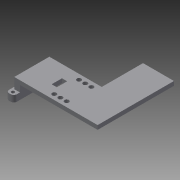
# Autodesk Inventor part: CartServoMountV2
Saved by Autodesk Inventor 2015 (Build 190159000, 159)
## iProperties
Created: 2016-03-28
Part Number: CartServoMountV2
Material: Generic
Document SubType Name: Modeling
Designer: Hatch
Density: 1 g/cm^3
Appearance: Default
Author: Hatch
Autodesk Inventor part; units mm, degrees
ref_plane "YZ Plane" through (0, 0, 0) normal (1, 0, 0) x (0, 1, 0)
ref_plane "XZ Plane" through (0, 0, 0) normal (0, 1, 0) x (-1, 0, 0)
ref_plane "XY Plane" through (0, 0, 0) normal (0, 0, 1) x (1, 0, 0)
sketch "Sketch1" plane through (0, 0, 0) normal (0, 1, 0) x (-1, 0, 0)
  line L0 (0, 0) -> (22, 0)
  line L1 (22, 0) -> (22, -34)
  line L2 (22, -34) -> (0, -34)
  line L3 (0, -34) -> (0, 0)
  dimension "d0" = 22
  dimension "d1" = 34
  constraints: 8 end point, 2 parallel, 1 horizontal, 1 perpendicular
  measures "d0" distance of L1.end L2.end
  measures "d1" distance of L0.end L1.end
extrude "Extrusion1" add sketch "Sketch1" along normal blind 4
sketch "Sketch2" plane through (0, 4, 0) normal (0, 1, 0) x (1, 0, 0)
  line L0 (-22, 0) -> (0, 0) projected
  circle A0 centre (-5, 5) radius 2.125
  dimension "d7" = 4.25
  constraints: 1 centre point
  measures "d7" diameter of A0
extrude "Extrusion2" cut sketch "Sketch2" against normal through all
pattern_linear "Rectangular Pattern1" count 3 spacing 6 along (-1, 0, 0) count 2 spacing 24 along (0, 0, -1) of "Extrusion2"
sketch "Sketch3" plane through (-22, 0, -34) normal (-1, 0, 0) x (0, 0, 1)
  line L0 (34, 0) -> (0, 0)
  line L1 (0, 0) -> (0, 4)
  line L2 (0, 4) -> (34, 4)
  line L3 (34, 4) -> (34, 0)
  constraints: 8 end point, 2 parallel, 1 horizontal, 1 perpendicular
extrude "Extrusion3" add sketch "Sketch3" along normal blind 23.25
sketch "Sketch4" plane through (0, 4, 0) normal (0, 1, 0) x (1, 0, 0)
  line L0 (-45.25, 0) -> (-50.75, 0)
  line L1 (-50.75, 0) -> (-50.75, 34)
  line L2 (-50.75, 34) -> (-45.25, 34)
  line L3 (-45.25, 34) -> (-45.25, 0)
  point P0 (0, 0)
  dimension "d18" = 5.5
  constraints: 8 end point, 2 parallel, 1 horizontal, 1 perpendicular
  measures "d18" distance of L1.end L2.end
extrude "Extrusion4" add sketch "Sketch4" against normal blind 16.5
sketch "Sketch5" plane through (-50.75, 4, -34) normal (-1, 0, 0) x (0, 0, 1)
  line L0 (0, -4) -> (0, -16.5) projected
  line L1 (34, -16.5) -> (0, -16.5)
  line L2 (0, -16.5) -> (0, -10.25)
  line L3 (0, -10.25) -> (34, -10.25)
  line L4 (34, -10.25) -> (34, -16.5)
  point P0 (34, -4)
  dimension "d21" = 6.25
  constraints: 8 end point, 2 parallel, 1 horizontal, 1 midpoint, 1 perpendicular
  measures "d21" distance of L1.end L2.end
extrude "Extrusion5" add sketch "Sketch5" along normal blind 2
sketch "Sketch6" plane through (0, 0, -34) normal (0, 0, -1) x (-1, 0, 0)
  line L0 (52.75, -6.25) -> (45.25, -6.25)
  line L1 (45.25, -6.25) -> (45.25, -12.5)
  line L2 (45.25, -12.5) -> (52.75, -12.5)
  line L3 (52.75, -12.5) -> (52.75, -6.25)
  point P0 (0, 0)
  constraints: 8 end point, 2 parallel, 1 horizontal, 1 perpendicular
extrude "Extrusion6" add sketch "Sketch6" along normal blind 6
sketch "Sketch7" plane through (0, 0, 0) normal (0, 0, 1) x (1, 0, 0)
  line L0 (-52.75, -12.5) -> (-45.25, -12.5)
  line L1 (-45.25, -12.5) -> (-45.25, -6.25)
  line L2 (-45.25, -6.25) -> (-52.75, -6.25)
  line L3 (-52.75, -6.25) -> (-52.75, -12.5)
  point P0 (0, 0)
  constraints: 8 end point, 2 parallel, 1 horizontal, 1 perpendicular
extrude "Extrusion7" add sketch "Sketch7" along normal blind 6
fillet "Fillet1" radius 3 1 edges at (-52.75, -9.375, 6)
fillet "Fillet2" radius 3 1 edges at (-45.25, -9.375, 6)
fillet "Fillet3" radius 3 1 edges at (-52.75, -9.375, -40)
fillet "Fillet4" radius 3 1 edges at (-45.25, -9.375, -40)
sketch "Sketch8" plane through (0, -12.5, 0) normal (0, -1, 0) x (1, 0, 0)
  line L0 (-45.25, -34) -> (-52.75, -34)
  line L1 (-52.75, 3) -> (-52.75, -37) projected
  line L2 (-45.25, -34) -> (0, -34) projected
  line L3 (-49.75, -40) -> (-48.25, -40) projected
  line L4 (-49, -40) -> (-49, -34)
  line L5 (-45.25, -34) -> (-50.75, -34) projected
  line L6 (-52.75, 0) -> (-45.25, 0)
  line L7 (-50.75, 0) -> (-45.25, 0) projected
  line L8 (-49.75, 6) -> (-48.25, 6) projected
  line L9 (-49, 6) -> (-49, 0)
  circle A0 centre (-49, -37) radius 1.5
  circle A1 centre (-49, 3) radius 1.5
  point P0 (0, 0)
  dimension "d32" = 3
  dimension "d33" = 3
  constraints: 8 end point, 4 midpoint, 4 point on line, 2 centre point, 2 collinear, 2 perpendicular
  measures "d32" diameter of A0
  measures "d33" diameter of A1
extrude "Extrusion8" cut sketch "Sketch8" against normal through all
sketch "Sketch9" plane through (0, 4, 0) normal (0, 1, 0) x (1, 0, 0)
  line L0 (0, 0) -> (0, 34) projected
  line L1 (0, 17) -> (-24, 17)
  line L2 (-21.5, 12) -> (-26.5, 12)
  line L3 (-26.5, 12) -> (-26.5, 22)
  line L4 (-26.5, 22) -> (-21.5, 22)
  line L5 (-21.5, 22) -> (-21.5, 12)
  line L6 (-21.5, 12) -> (-26.5, 22) construction
  line L7 (-26.5, 12) -> (-21.5, 22) construction
  dimension "d36" = 24
  dimension "d37" = 5
  dimension "d38" = 10
  constraints: 14 end point, 3 midpoint, 2 horizontal, 2 parallel, 1 perpendicular
  measures "d36" distance of L1.start L1.end
  measures "d37" distance of L3.end L4.end
  measures "d38" distance of L2.end L3.end
extrude "Extrusion9" cut sketch "Sketch9" against normal through all
sketch "Sketch10" plane through (0, 0, 0) normal (1, 0, 0) x (0, 0, -1)
  line L0 (0, 4) -> (34, 4)
  line L1 (34, 4) -> (34, 0)
  line L2 (34, 0) -> (0, 0)
  line L3 (0, 0) -> (0, 4)
  constraints: 8 end point, 2 parallel, 1 horizontal, 1 perpendicular
extrude "Extrusion10" add sketch "Sketch10" along normal blind 30
sketch "Sketch11" plane through (-45.25, -6.25, -34) normal (0, 0, -1) x (-1, 0, 0)
  line L0 (-75.25, 10.25) -> (-45.25, 10.25)
  line L1 (-45.25, 10.25) -> (-45.25, 6.25)
  line L2 (-45.25, 6.25) -> (-75.25, 6.25)
  line L3 (-75.25, 6.25) -> (-75.25, 10.25)
  constraints: 8 end point, 2 parallel, 1 horizontal, 1 perpendicular
extrude "Extrusion11" add sketch "Sketch11" along normal blind 40
body "Solid1"
